Autodesk Inventor part; units mm, degrees
(part 3 of 3)
extrude "Extrusion7" cut sketch "Sketch7" against normal blind 10 contours A1 L6 A2 L5 | L8 A4 L9 A3 | A6 L13 A5 L12 | L15 A7 L17 A8 | A10 L20 A9 L19 | L22 A11 L24 A12 | A14 L27 A13 L26 | L29 A15 L31 A16 | A18 L34 A17 L33 | L36 A19 L38 A20 | A22 L41 A21 L40 | L43 A23 L45 A24 | A26 L48 A25 L47 | L50 A27 L52 A28 | A30 L55 A29 L54 | L57 A31 L59 A32 | A46 L83 A45 L82 | L85 A47 L87 A48 | A50 L90 A49 L89 | L92 A51 L94 A52 | A54 L97 A53 L96 | L99 A55 L101 A56 | A58 L104 A57 L103 | L106 A59 L108 A60 | A62 L111 A61 L110 | L113 A63 L115 A64 | A66 L118 A65 L117 | L120 A67 L122 A68 | A70 L125 A69 L124 | L127 A71 L129 A72 | A74 L132 A73 L131 | L134 A75 L136 A76 | A78 L139 A77 L138 | L141 A79 L143 A80 | A90 L160 A89 L159 | L162 A91 L164 A92 | A94 L167 A93 L166 | L169 A95 L171 A96 | A98 L174 A97 L173 | L176 A99 L178 A100 | A102 L181 A101 L180 | L183 A103 L185 A104 | A106 L188 A105 L187 | L190 A107 L192 A108 | A110 L195 A109 L194 | L197 A111 L199 A112 | A114 L202 A113 L201 | L204 A115 L206 A116 | A118 L209 A117 L208 | L211 A119 L213 A120 | A122 L216 A121 L215 | L218 A123 L220 A124 | A126 L223 A125 L222 | L225 A127 L227 A128 | A134 L237 A133 L236 | L239 A135 L241 A136 | A138 L244 A137 L243 | L246 A139 L248 A140 | A142 L251 A141 L250 | L253 A143 L255 A144 | A146 L258 A145 L257 | L260 A147 L262 A148 | A150 L265 A149 L264 | L267 A151 L269 A152 | A154 L272 A153 L271 | L274 A155 L276 A156 | A158 L279 A157 L278 | L281 A159 L283 A160 | A162 L286 A161 L285 | L288 A163 L290 A164 | A166 L293 A165 L292 | L295 A167 L297 A168 | A170 L300 A169 L299 | L302 A171 L304 A172 | A174 L307 A173 L306 | L309 A175 L311 A176 | A178 L314 A177 L313 | L316 A179 L318 A180 | A182 L321 A181 L320 | L323 A183 L325 A184 | A186 L328 A185 L327 | L330 A187 L332 A188 | A190 L335 A189 L334 | L337 A191 L339 A192 | A194 L342 A193 L341 | L344 A195 L346 A196 | A198 L349 A197 L348 | L351 A199 L353 A200 | A202 L356 A201 L355 | L358 A203 L360 A204 | A206 L363 A205 L362 | L365 A207 L367 A208 | A210 L370 A209 L369 | L372 A211 L374 A212 | A214 L377 A213 L376 | L379 A215 L381 A216 | A218 L384 A217 L383 | L386 A219 L388 A220 | A222 L391 A221 L390 | L393 A223 L395 A224 | A226 L398 A225 L397 | L400 A227 L402 A228 | A230 L405 A229 L404 | L407 A231 L409 A232 | A234 L412 A233 L411 | L414 A235 L416 A236 | A238 L419 A237 L418 | L421 A239 L423 A240 | A242 L426 A241 L425 | L428 A243 L430 A244 | A246 L433 A245 L432 | L435 A247 L437 A248 | A250 L440 A249 L439 | L442 A251 L444 A252 | A254 L447 A253 L446 | L449 A255 L451 A256 | A258 L454 A257 L453 | L456 A259 L458 A260 | A262 L461 A261 L460 | L463 A263 L465 A264 | A266 L468 A265 L467 | L470 A267 L472 A268 | A270 L475 A269 L474 | L477 A271 L479 A272 | A274 L482 A273 L481 | L484 A275 L486 A276 | A278 L489 A277 L488 | L491 A279 L493 A280 | A282 L496 A281 L495 | L498 A283 L500 A284 | A286 L503 A285 L502 | L505 A287 L507 A288 | A290 L510 A289 L509 | L512 A291 L514 A292 | A294 L517 A293 L516 | L519 A295 L521 A296 | A298 L524 A297 L523 | L526 A299 L528 A300 | A302 L531 A301 L530 | L533 A303 L535 A304 | A306 L538 A305 L537 | L540 A307 L542 A308 | A310 L545 A309 L544 | L547 A311 L549 A312 | A314 L552 A313 L551 | L554 A315 L556 A316 | A318 L559 A317 L558 | L561 A319 L563 A320 | A322 L566 A321 L565 | L568 A323 L570 A324 | A326 L573 A325 L572 | L575 A327 L577 A328 | A330 L580 A329 L579 | L582 A331 L584 A332 | A334 L587 A333 L586 | L589 A335 L591 A336 | A338 L594 A337 L593 | L596 A339 L598 A340 | A342 L601 A341 L600 | L603 A343 L605 A344 | A346 L608 A345 L607 | L610 A347 L612 A348 | A350 L615 A349 L614 | L617 A351 L619 A352 | A354 L622 A353 L621 | L624 A355 L626 A356 | A358 L629 A357 L628 | L631 A359 L633 A360 | A362 L636 A361 L635 | L638 A363 L640 A364 | A366 L643 A365 L642 | L645 A367 L647 A368 | A370 L650 A369 L649 | L652 A371 L654 A372 | A374 L657 A373 L656 | L659 A375 L661 A376 | A378 L664 A377 L663 | L666 A379 L668 A380 | A382 L671 A381 L670 | L673 A383 L675 A384 | A386 L678 A385 L677 | L680 A387 L682 A388 | A390 L685 A389 L684 | L687 A391 L689 A392 | A394 L692 A393 L691 | L694 A395 L696 A396 | A398 L699 A397 L698 | L701 A399 L703 A400 | A402 L706 A401 L705 | L708 A403 L710 A404 | A406 L713 A405 L712 | L715 A407 L717 A408 | A410 L720 A409 L719 | L722 A411 L724 A412 | A414 L727 A413 L726 | L729 A415 L731 A416 | A418 L734 A417 L733 | L736 A419 L738 A420 | A422 L741 A421 L740 | L743 A423 L745 A424 | A426 L748 A425 L747 | L750 A427 L752 A428 | A430 L755 A429 L754 | L757 A431 L759 A432 | A434 L762 A433 L761 | L764 A435 L766 A436 | A438 L769 A437 L768 | L771 A439 L773 A440 | A442 L776 A441 L775 | L778 A443 L780 A444 | A446 L783 A445 L782 | L785 A447 L787 A448 | A450 L790 A449 L789 | L792 A451 L794 A452 | A454 L797 A453 L796 | L799 A455 L801 A456 | A458 L804 A457 L803 | L806 A459 L808 A460 | A462 L811 A461 L810 | L813 A463 L815 A464 | A466 L818 A465 L817 | L820 A467 L822 A468 | A470 L825 A469 L824 | L827 A471 L829 A472 | A474 L832 A473 L831 | L834 A475 L836 A476 | A478 L839 A477 L838 | L841 A479 L843 A480 | A482 L846 A481 L845 | L848 A483 L850 A484
sketch "Sketch8" plane through (3, 0, 0) normal (1, 0, 0) x (0, 0, -1)
  arc A0 (170, 157) -> (157, 170) centre (157, 157) ccw projected
  circle A1 centre (147, 147) radius 8
  line L0 (157, 157) -> (147, 147) construction
  line L1 (170, 0) -> (170, 157) projected
  point P0 (0, 0)
  dimension "d114" = 16
  dimension "d115" = 45
  dimension "d116" = 10
  constraints: 2 end point, 1 centre point
  measures "d114" diameter of A1
  measures "d115" angle of L1 L0
  measures "d116" horizontal distance of L0.start L0.end
extrude "Extrusion8" cut sketch "Sketch8" against normal blind 10
body "Solid1"
